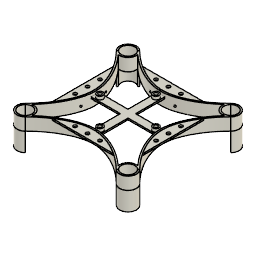
drone_v0-03_frame (Autodesk Fusion 360 design; units mm, degrees)
Autodesk Fusion 360 part; units mm, degrees
sketch "スケッチ1" plane through (0, 0, 0) normal (0, 0, 1) x (1, 0, 0)
  line L0 (-86.2009, 0) -> (97.1816, 0) construction
  line L1 (0, 73.8215) -> (0, -82.3449) construction
  circle A0 centre (-33, 33) radius 4.35
  line L2 (-58.834, 58.834) -> (93.8083, -93.8083) construction
  line L3 (-53.1247, 33) -> (-9.7608, 33) construction
  line L4 (-44.9526, 21.0474) -> (-18.1811, 47.8189) construction
  circle A1 centre (-18, 0) radius 1.1
  circle A2 centre (-18, 0) radius 2
  line L5 (-26, 10) -> (-26, -10.1107) construction
  circle A3 centre (-26, 0) radius 1.1
  circle A4 centre (-26, 8) radius 1.1
  line L6 (-33.6275, 28.6955) -> (-28.6955, 33.6275)
  circle A5 centre (-38.9397, 38.9397) radius 1.1
  line L7 (-37.3045, 32.3725) -> (-32.3725, 37.3045)
  circle A6 centre (-26, -8) radius 1.1
  line L8 (-47.3501, 29.062) -> (-51.4513, 24.9608)
  line L9 (-54.6333, 28.1428) -> (-50.5321, 32.244)
  line L10 (-51.4513, 24.9608) -> (-54.6333, 28.1428)
  line L11 (-50.5321, 32.244) -> (-47.3501, 29.062)
  circle A7 centre (-38.9397, -38.9397) radius 1.1
  circle A8 centre (-33, -33) radius 4.35
  line L12 (-32.3725, -37.3045) -> (-37.3045, -32.3725)
  line L13 (-28.6955, -33.6275) -> (-33.6275, -28.6955)
  circle A9 centre (0, -18) radius 1.1
  circle A10 centre (0, -18) radius 2
  circle A11 centre (0, -26) radius 1.1
  circle A12 centre (8, -26) radius 1.1
  circle A13 centre (-8, -26) radius 1.1
  circle A14 centre (38.9397, -38.9397) radius 1.1
  circle A15 centre (33, -33) radius 4.35
  line L14 (37.3045, -32.3725) -> (32.3725, -37.3045)
  line L15 (33.6275, -28.6955) -> (28.6955, -33.6275)
  circle A16 centre (18, 0) radius 1.1
  circle A17 centre (18, 0) radius 2
  circle A18 centre (26, 0) radius 1.1
  circle A19 centre (26, 8) radius 1.1
  circle A20 centre (26, -8) radius 1.1
  circle A21 centre (38.9397, 38.9397) radius 1.1
  circle A22 centre (33, 33) radius 4.35
  line L16 (32.3725, 37.3045) -> (37.3045, 32.3725)
  line L17 (28.6955, 33.6275) -> (33.6275, 28.6955)
  circle A23 centre (0, 18) radius 1.1
  circle A24 centre (0, 18) radius 2
  circle A25 centre (0, 26) radius 1.1
  circle A26 centre (-8, 26) radius 1.1
  circle A27 centre (8, 26) radius 1.1
  line L18 (-50.5321, 32.244) -> (-51.4513, 24.9608) construction
  line L19 (-47.3501, 29.062) -> (-54.6333, 28.1428) construction
  circle A28 centre (-38.9397, 27.0603) radius 1.1
  circle A29 centre (-27.0603, 38.9397) radius 1.1
  circle A30 centre (-38.9397, -27.0603) radius 1.1
  circle A31 centre (-27.0603, -38.9397) radius 1.1
  circle A32 centre (27.0603, -38.9397) radius 1.1
  circle A33 centre (38.9397, -27.0603) radius 1.1
  circle A34 centre (38.9397, 27.0603) radius 1.1
  circle A35 centre (27.0603, 38.9397) radius 1.1
  point P0 (-22, 0)
  point P1 (-50.9917, 28.6024)
  dimension "md" = 8.7
  dimension "d3" = 8.7
  dimension "d4" = 33
  dimension "d5" = 33
  dimension "d6" = 45
  dimension "d7" = 2.2
  dimension "d8" = 4
  dimension "d9" = 18
  dimension "d10" = 22
  dimension "d11" = 4
  dimension "d12" = 2.2
  dimension "d13" = 2.2
  dimension "d14" = 8
  dimension "d15" = 2.6
  dimension "d16" = 2.2
  dimension "d18" = 5.8
  dimension "d19" = 4.5
  dimension "d21" = 360
  dimension "d106" = 8.4
  dimension "d115" = 2.2
  dimension "d116" = 8.4
  dimension "d118" = 360
  constraint horizontal L0
  constraint vertical L1
  constraint coincident origin L0
  constraint coincident origin L1
  constraint coincident origin L2
  constraint coincident A0.centre L2
  constraint horizontal L3
  constraint coincident A0.centre L3
  constraint coincident A0.centre L4
  constraint coincident L0 A1.centre
  constraint concentric A1 A2
  constraint coincident L0 P0
  constraint vertical L5
  constraint coincident L5 A3.centre
  constraint coincident L0 A3.centre
  constraint coincident L5 A4.centre
  constraint coincident A0 L6.start
  constraint coincident A0 L6.end
  constraint parallel L4 L6
  constraint coincident L2 A5.centre
  constraint symmetric L4 L6.start L7.start
  constraint symmetric L4 L6.end L7.end
  constraint symmetric L0 A4 A6
  constraint perpendicular L8 L11
  constraint perpendicular L8 L10
  constraint perpendicular L9 L10
  constraint midpoint L19 P1
  constraint coincident L4 A28.centre
  constraint symmetric L2 A28 A29
  measures "d3" diameter of A0
  measures "d4" distance of L1 A0.centre
  measures "d5" distance of L0 A0.centre
  measures "d6" angle of L3 L4
  measures "d7" diameter of A1
  measures "d8" diameter of A2
  measures "d9" distance of L1 A1.centre
  measures "d10" distance of L1 P0
  measures "d11" distance of P0 L5
  measures "d12" diameter of A3
  measures "d13" diameter of A4
  measures "d14" distance of L0 A4.centre
  measures "d15" distance of L4 L6
  measures "d16" diameter of A5
  measures "d18" distance of L8.end L8.start
  measures "d19" distance of L9.end L8.start
  measures "d106" distance of A0.centre A5.centre
  measures "d115" diameter of A28
  measures "d116" distance of A0.centre A28.centre
sketch "スケッチ2" plane through (0, 0, 0) normal (0, 0, 1) x (1, 0, 0)
  line L0 (-60, 0) -> (65.9747, 0) construction
  line L1 (0, 60) -> (0, -54.7392) construction
  circle A0 centre (-33, 33) radius 5.35
  line L2 (-57.7718, 57.7718) -> (84.0395, -84.0395) construction
  circle A1 centre (-33, -33) radius 5.35
  circle A2 centre (33, -33) radius 5.35
  circle A3 centre (33, 33) radius 5.35
  spline S0 degree 5 poles (-29.217, 36.783) (-28.1363, 35.7024) (-25.9271, 33.6247) (-22.4702, 30.759) (-17.6335, 27.4601) (-11.5151, 24.3277) (-5.5833, 22.3445) (0, 21.658) (5.5834, 22.3445) (11.5151, 24.3277) (17.6335, 27.4601) (22.4702, 30.759) (25.9271, 33.6247) (28.1363, 35.7024) (29.217, 36.783) knots 0 0 0 0 0 0 0.1 0.2 0.3 0.4 0.5 0.6 0.7 0.8 0.9 1 1 1 1 1 1
  line L3 (-5, 22) -> (5, 22)
  line L4 (-34.1667, 41.7328) -> (-24.2672, 31.8333)
  line L5 (24.2672, 31.8333) -> (34.1667, 41.7328)
  line L6 (-29, 21.4643) -> (-29, -21.4643)
  spline S1 degree 3 poles (-29.9241, 36.0759) (-25.5902, 31.742) (-20.7348, 28.1691) (-15.8501, 25.5622) (-11.9177, 23.4636) (-8.0143, 22.0048) (-4.2565, 21.3664) (-0.3531, 20.7034) (3.4515, 20.9635) (7.422, 22.0866) (12.3159, 23.4709) (17.4778, 26.1112) (22.387, 29.6525) (25.0074, 31.5428) (27.5398, 33.6917) (29.9241, 36.0759) knots 0 0 0 0 0.23685 0.23685 0.23685 0.427521 0.427521 0.427521 0.625581 0.625581 0.625581 0.869698 0.869698 0.869698 1 1 1 1
  spline S2 degree 5 poles (-36.783, -29.217) (-35.7024, -28.1363) (-33.6247, -25.9271) (-30.759, -22.4702) (-27.4601, -17.6335) (-24.3277, -11.5151) (-22.3445, -5.5833) (-21.658, 0) (-22.3445, 5.5834) (-24.3277, 11.5151) (-27.4601, 17.6335) (-30.759, 22.4702) (-33.6247, 25.9271) (-35.7024, 28.1363) (-36.783, 29.217) knots 0 0 0 0 0 0 0.1 0.2 0.3 0.4 0.5 0.6 0.7 0.8 0.9 1 1 1 1 1 1
  spline S3 degree 3 poles (-36.0759, -29.9241) (-31.742, -25.5902) (-28.1691, -20.7348) (-25.5622, -15.8501) (-23.4636, -11.9177) (-22.0048, -8.0143) (-21.3664, -4.2565) (-20.7034, -0.3531) (-20.9635, 3.4515) (-22.0866, 7.422) (-23.4709, 12.3159) (-26.1112, 17.4778) (-29.6525, 22.387) (-31.5428, 25.0074) (-33.6917, 27.5398) (-36.0759, 29.9241) knots 0 0 0 0 0.23685 0.23685 0.23685 0.427521 0.427521 0.427521 0.625581 0.625581 0.625581 0.869698 0.869698 0.869698 1 1 1 1
  spline S4 degree 5 poles (29.217, -36.783) (28.1363, -35.7024) (25.9271, -33.6247) (22.4702, -30.759) (17.6335, -27.4601) (11.5151, -24.3277) (5.5833, -22.3445) (0, -21.658) (-5.5834, -22.3445) (-11.5151, -24.3277) (-17.6335, -27.4601) (-22.4702, -30.759) (-25.9271, -33.6247) (-28.1363, -35.7024) (-29.217, -36.783) knots 0 0 0 0 0 0 0.1 0.2 0.3 0.4 0.5 0.6 0.7 0.8 0.9 1 1 1 1 1 1
  spline S5 degree 3 poles (29.9241, -36.0759) (25.5902, -31.742) (20.7348, -28.1691) (15.8501, -25.5622) (11.9177, -23.4636) (8.0143, -22.0048) (4.2565, -21.3664) (0.3531, -20.7034) (-3.4515, -20.9635) (-7.422, -22.0866) (-12.3159, -23.4709) (-17.4778, -26.1112) (-22.387, -29.6525) (-25.0074, -31.5428) (-27.5398, -33.6917) (-29.9241, -36.0759) knots 0 0 0 0 0.23685 0.23685 0.23685 0.427521 0.427521 0.427521 0.625581 0.625581 0.625581 0.869698 0.869698 0.869698 1 1 1 1
  spline S6 degree 5 poles (36.783, 29.217) (35.7024, 28.1363) (33.6247, 25.9271) (30.759, 22.4702) (27.4601, 17.6335) (24.3277, 11.5151) (22.3445, 5.5833) (21.658, 0) (22.3445, -5.5834) (24.3277, -11.5151) (27.4601, -17.6335) (30.759, -22.4702) (33.6247, -25.9271) (35.7024, -28.1363) (36.783, -29.217) knots 0 0 0 0 0 0 0.1 0.2 0.3 0.4 0.5 0.6 0.7 0.8 0.9 1 1 1 1 1 1
  spline S7 degree 3 poles (36.0759, 29.9241) (31.742, 25.5902) (28.1691, 20.7348) (25.5622, 15.8501) (23.4636, 11.9177) (22.0048, 8.0143) (21.3664, 4.2565) (20.7034, 0.3531) (20.9635, -3.4515) (22.0866, -7.422) (23.4709, -12.3159) (26.1112, -17.4778) (29.6525, -22.387) (31.5428, -25.0074) (33.6917, -27.5398) (36.0759, -29.9241) knots 0 0 0 0 0.23685 0.23685 0.23685 0.427521 0.427521 0.427521 0.625581 0.625581 0.625581 0.869698 0.869698 0.869698 1 1 1 1
  arc A4 (-29.9241, 36.0759) -> (-36.0759, 29.9241) centre (-33, 33) ccw
  arc A5 (-36.0759, -29.9241) -> (-29.9241, -36.0759) centre (-33, -33) ccw
  arc A6 (29.9241, -36.0759) -> (36.0759, -29.9241) centre (33, -33) ccw
  arc A7 (36.0759, 29.9241) -> (29.9241, 36.0759) centre (33, 33) ccw
  line L7 (-36.783, 29.217) -> (-36.0759, 29.9241)
  line L8 (-29.9241, 36.0759) -> (-29.217, 36.783)
  point P0 (0, 22)
  point P1 (0, 22)
  point P2 (-22, 0)
  point P3 (0, -22)
  point P4 (22, 0)
  dimension "d22" = 10.7
  dimension "d23" = 33
  dimension "d24" = 33
  dimension "d25" = 22
  dimension "d28" = 10
  dimension "d29" = 14
  dimension "d30" = 14
  dimension "d35" = 29
  dimension "d193" = 1
  dimension "d195" = 360
  dimension "d197" = 360
  constraint horizontal L0
  constraint vertical L1
  constraint coincident origin L0
  constraint coincident origin L1
  constraint coincident L1 P1
  constraint coincident A0.centre L2
  constraint coincident origin L2
  constraint coincident A0 S0.start
  constraint coincident P1 P0
  constraint coincident A3 S0.end
  constraint midpoint P1 L3
  constraint horizontal L3
  constraint midpoint S0.start L4
  constraint midpoint S0.end L5
  constraint parallel L2 L4
  constraint symmetric L1 L4 L5
  constraint vertical L6
  constraint tangent A0 S0
  constraint tangent A3 S0
  constraint coincident L6.start S3
  constraint coincident L6.end S3
  measures "d22" diameter of A0
  measures "d23" distance of L1 A0.centre
  measures "d24" distance of L0 A0.centre
  measures "d25" distance of L0 P1
  measures "d28" distance of L3.start L3.end
  measures "d29" distance of L4.start L4.end
  measures "d30" distance of L5.start L5.end
  measures "d35" distance of L1 L6
ref_plane "作業平面1" through (0, 0, -2) normal (0, 0, 1) x (1, 0, 0)
sketch "スケッチ3" plane through (0, 0, -2) normal (0, 0, 1) x (1, 0, 0)
  line L0 (-78.648, 0) -> (80, 0) construction
  line L1 (0, 70) -> (0, -68.6125) construction
  line L2 (-2.5, 21.5) -> (-2.5, 2.5)
  line L3 (-2.5, 2.5) -> (-21.5, 2.5)
  line L4 (-2.5, -2.5) -> (-2.5, -21.5)
  line L5 (-21.5, -2.5) -> (-2.5, -2.5)
  line L6 (2.5, -2.5) -> (21.5, -2.5)
  line L7 (2.5, -21.5) -> (2.5, -2.5)
  line L8 (2.5, 2.5) -> (2.5, 21.5)
  line L9 (21.5, 2.5) -> (2.5, 2.5)
  line L10 (-21.5, 2.5) -> (-21.5, -2.5)
  line L11 (-2.5, -21.5) -> (2.5, -21.5)
  line L12 (21.5, -2.5) -> (21.5, 2.5)
  line L13 (2.5, 21.5) -> (-2.5, 21.5)
  dimension "d38" = 2.5
  dimension "d39" = 2.5
  dimension "d40" = 19
  dimension "d41" = 19
  dimension "d43" = 360
  dimension "d45" = 360
  constraint horizontal L0
  constraint vertical L1
  constraint coincident origin L0
  constraint coincident origin L1
  constraint vertical L2
  constraint perpendicular L2 L3
  measures "d38" distance of L1 L2
  measures "d39" distance of L0 L3
  measures "d40" distance of L2.end L3.end
  measures "d41" distance of L2.start L2.end
ref_plane "作業平面2" through (0, 0, 12.125) normal (0.707107, 0.707107, 0) x (0, 0, 1)
ref_plane "作業平面3" through (0, 0, 12.125) normal (-0.707107, 0.707107, 0) x (0, 0, 1)
sketch "スケッチ4" plane through (0, 0, 0) normal (0, 1, 0) x (1, 0, 0)
  line L0 (0, -32.7268) -> (0, 60) construction
  line L1 (-31.6399, 5) -> (37.1122, 5) construction
  line L2 (-9.2, 8) -> (9.2, 8)
  line L3 (9.2, 8) -> (9.2, 16)
  line L4 (9.2, 16) -> (-9.2, 16)
  line L5 (-9.2, 16) -> (-9.2, 8)
  circle A0 centre (0, 5) radius 0.6
  circle A1 centre (8, 5) radius 0.6
  circle A2 centre (-8, 5) radius 0.6
  dimension "d48" = 5
  dimension "d49" = 8
  dimension "d50" = 8
  dimension "d51" = 9.2
  dimension "d52" = 9.2
  dimension "d53" = 1.2
  dimension "d54" = 1.2
  dimension "d56" = 8
  constraint vertical L0
  constraint coincident origin L0
  constraint horizontal L1
  constraint horizontal L2
  constraint vertical L3
  constraint horizontal L4
  constraint vertical L5
  constraint coincident L1 A0.centre
  constraint coincident L0 A0.centre
  constraint coincident L1 A1.centre
  constraint symmetric L0 A1 A2
  measures "d48" distance of origin L1
  measures "d49" distance of L2.end L3.end
  measures "d50" distance of origin L2
  measures "d51" distance of L0 L3
  measures "d52" distance of L0 L5
  measures "d53" diameter of A0
  measures "d54" diameter of A1
  measures "d56" distance of L0 A1.centre
sketch "スケッチ5" plane through (0, 0, 0) normal (1, 0, 0) x (0, 1, 0)
  line L0 (0, 10.0554) -> (0, -26.1679) construction
  line L1 (-11.7872, -5) -> (12.0114, -5) construction
  line L2 (-9.2, -8) -> (9.2, -8)
  line L3 (9.2, -8) -> (9.2, -16)
  line L4 (9.2, -16) -> (-9.2, -16)
  line L5 (-9.2, -16) -> (-9.2, -8)
  circle A0 centre (0, -5) radius 0.6
  circle A1 centre (8, -5) radius 0.6
  circle A2 centre (-8, -5) radius 0.6
  dimension "d57" = 5
  dimension "d58" = 8
  dimension "d59" = 8
  dimension "d60" = 9.2
  dimension "d61" = 9.2
  dimension "d62" = 1.2
  dimension "d63" = 1.2
  dimension "d64" = 8
  constraint vertical L0
  constraint coincident origin L0
  constraint horizontal L1
  constraint horizontal L2
  constraint vertical L3
  constraint horizontal L4
  constraint vertical L5
  constraint coincident L1 A0.centre
  constraint coincident L0 A0.centre
  constraint coincident L1 A1.centre
  constraint symmetric L0 A1 A2
  measures "d57" distance of origin L1
  measures "d58" distance of L2.end L3.end
  measures "d59" distance of origin L2
  measures "d60" distance of L0 L3
  measures "d61" distance of L0 L5
  measures "d62" diameter of A0
  measures "d63" diameter of A1
  measures "d64" distance of L0 A1.centre
sketch "スケッチ9" plane through (0, 0, 0) normal (0, 0, 1) x (1, 0, 0)
  line L0 (-120, 0) -> (66.0422, 0) construction
  line L1 (0, 70.4511) -> (0, -54.343) construction
  line L2 (-50.1244, 50.1244) -> (83.7076, -83.7076) construction
  line L3 (-40.4953, 37.3841) -> (-37.7857, 34.6744)
  line L4 (-34.6744, 37.7857) -> (-37.3841, 40.4953)
  arc A0 (-37.3841, 40.4953) -> (-40.4953, 37.3841) centre (-38.9397, 38.9397) ccw
  line L5 (-37.7857, 34.6744) -> (-34.6744, 37.7857)
  line L6 (-37.3841, 25.5047) -> (-34.6744, 28.2143)
  arc A1 (-40.4953, 28.6159) -> (-37.3841, 25.5047) centre (-38.9397, 27.0603) ccw
  line L7 (-37.7857, 31.3256) -> (-40.4953, 28.6159)
  line L8 (-34.6744, 28.2143) -> (-37.7857, 31.3256)
  line L9 (-28.6159, 40.4953) -> (-31.3256, 37.7857)
  arc A2 (-25.5047, 37.3841) -> (-28.6159, 40.4953) centre (-27.0603, 38.9397) ccw
  line L10 (-28.2143, 34.6744) -> (-25.5047, 37.3841)
  line L11 (-31.3256, 37.7857) -> (-28.2143, 34.6744)
  arc A3 (-28.0515, 39.2859) -> (-39.2579, 28.0162) centre (-33, 33) ccw
  arc A4 (-31.1073, 38.004) -> (-38.004, 31.1073) centre (-33, 33) ccw
  point P0 (-33, 33)
  dimension "d124" = 33
  dimension "d125" = 33
  dimension "d126" = 8.4
  dimension "d128" = 4.4
  dimension "d130" = 360
  dimension "d177" = 10.7
  dimension "d183" = 16
  constraint horizontal L0
  constraint coincident origin L0
  constraint vertical L1
  constraint coincident origin L1
  constraint coincident P0 L2
  constraint coincident origin L2
  constraint tangent L4 A0
  constraint tangent L3 A0
  constraint coincident L2 A0.centre
  constraint parallel L2 L3
  constraint parallel L2 L4
  constraint perpendicular L3 L5
  constraint coincident P0 A3.centre
  constraint coincident L9 A4.start
  constraint coincident L7 A4.end
  measures "d124" distance of L1 P0
  measures "d125" distance of L0 P0
  measures "d126" distance of P0 A0.centre
  measures "d128" diameter of A0
  measures "d177" diameter of A4
  measures "d183" diameter of A3
extrude "押し出し20" add sketch "スケッチ3" against normal blind 1 makes body 1
extrude "押し出し21" add sketch "スケッチ1" against normal blind 2 contours A2 | A10 | A17 | A24 bodies 1
extrude "押し出し22" cut sketch "スケッチ1" against normal blind 3 contours A1 | A9 | A16 | A23 bodies 1
extrude "押し出し32" add sketch "スケッチ9" against normal blind 1 separate body contours L3 L4 A3 A4 | L3 L7 A3 A4 | L4 L9 A3 A4 | L6 A1 L7 L8 | L9 A2 L10 L11 makes body 2
extrude "押し出し33" cut sketch "スケッチ1" against normal blind 1 contours A28 | A29 bodies 2
pattern_circular "C パターン7" count 4 over 360 about axis through (0, 0, 1.75) along (0, 0, 1) of bodies 2 makes body 3 at (-29.0434, -36.9372, 0) makes body 4 at (36.9372, -29.0434, 0) makes body 5 at (29.0434, 36.9372, 0)
extrude "押し出し35" add sketch "スケッチ2" against normal blind 1 separate body contours L6 S2 makes body 6
extrude "押し出し36" cut sketch "スケッチ1" against normal blind 1 contours A3 | A4 | A6 bodies 6
pattern_circular "C パターン10" count 4 over 360 about axis through (0, 0, 1.75) along (0, 0, 1) of bodies 6 makes body 7 at (4.0959, -24.6324, 0) makes body 8 at (24.6324, 4.0959, 0) makes body 9 at (-4.0959, 24.6324, 0)
extrude "押し出し37" add sketch "スケッチ2" against normal blind 8 separate body contours A0 A4 L7 L8 | A0 A3 S0 S1 | A0 S1 L8 | A0 S3 L7 makes body 10
extrude "押し出し38" cut sketch "スケッチ4" along normal blind 25 contours A0 | A1 | A2 bodies 10
pattern_circular "C パターン11" count 4 over 360 about axis through (0, 0, 1.75) along (0, 0, 1) of bodies 10 makes body 11 at (-32.158, -25.6221, -5.3333) makes body 12 at (23.4474, -30.4367, -5.3333) makes body 13 at (32.158, 25.6221, -2.6667)
combine "結合3" operation add target body 10 tool bodies 11 12 13
extrude "押し出し42" add sketch "スケッチ2" against normal blind 8 contours A0 S1 S3 A4 | A3 S1 S7 A7 | A2 S5 S7 A6 | A1 S3 S5 A5 picked at (31.6483, 31.8367) picked at (31.8367, -31.6483) picked at (-31.6744, -31.8071) bodies 10
extrude "押し出し43" cut sketch "スケッチ1" against normal blind 7 contours A0 L6 | A0 L6 L7 | A0 L7 | A8 L13 | A8 L12 L13 | A8 L12 | A15 L14 | A15 L14 L15 | A15 L15 | A22 L16 | A22 L16 L17 | A22 L17 bodies 10
extrude "押し出し44" cut sketch "スケッチ1" against normal blind 8 contours A0 L6 L7 | A8 L12 L13 | A15 L14 L15 | A22 L16 L17 bodies 10
extrude "押し出し45" add sketch "スケッチ2" against normal blind 20 separate body contours A0 A4 L7 L8 makes body 14
pattern_circular "C パターン14" count 4 over 360 about axis through (0, 0, 1.75) along (0, 0, 1) of bodies 14 makes body 15 at (-29.6125, -37.1409, -13.3333) makes body 16 at (37.1409, -29.6125, -13.3333) makes body 17 at (29.6125, 37.1409, -13.3333)
hidden bodies 2 3 4 5
equation "md = 8.7 mm"
equation "D = md + 2 mm"
equation "d3 = md"
equation "d22 = D"
equation "d177 = D"
